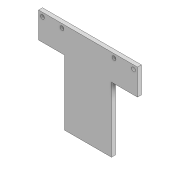
# Autodesk Inventor part: rotator_support
Saved by Autodesk Inventor 2020 (Build 240168000, 168)
## iProperties
Created: 2021-05-10
Part Number: rotator_support
Material: Generic
Document SubType Name: Modeling
Designer: Hsu Daniel
Density: 1 g/cm^3
Appearance: Default
Author: Hsu Daniel
Autodesk Inventor part; units mm, degrees
ref_plane "YZ Plane" through (0, 0, 0) normal (1, 0, 0) x (0, 1, 0)
ref_plane "XZ Plane" through (0, 0, 0) normal (0, 1, 0) x (-1, 0, 0)
ref_plane "XY Plane" through (0, 0, 0) normal (0, 0, 1) x (1, 0, 0)
sketch "Sketch1" plane through (0, 0, 0) normal (0, 0, 1) x (1, 0, 0)
  line L0 (0, 0) -> (0, 50)
  line L1 (0, 50) -> (-20, 50)
  line L2 (-20, 50) -> (-20, 70)
  line L3 (-20, 70) -> (18, 70)
  line L4 (18, 70) -> (18, 0) construction
  line L5 (18, 0) -> (0, 0)
  line L6 (36, 0) -> (36, 50)
  line L7 (36, 50) -> (56, 50)
  line L8 (56, 50) -> (56, 70)
  line L9 (56, 70) -> (18, 70)
  line L10 (18, 0) -> (36, 0)
  circle A0 centre (-17, 67) radius 1.5
  circle A1 centre (-2, 67) radius 1.5
  circle A2 centre (53, 67) radius 1.5
  circle A3 centre (38, 67) radius 1.5
  line L11 (-17, 67) -> (-20, 67) construction
  dimension "d1" = 20
  dimension "d2" = 20
  dimension "d3" = 36
  dimension "d4" = 70
  dimension "d5" = 3
  dimension "d6" = 3
  dimension "d7" = 15
  dimension "d8" = 3
  dimension "d9" = 3
  constraints: 24 end point, 6 perpendicular, 6 symmetric about line, 4 centre point, 2 point on line, 1 vertical, 2 other
  measures "d1" distance of L0.end L1.end
  measures "d2" distance of L1.end L2.end
  measures "d3" distance between parallel lines of L6 L0
  measures "d4" distance between parallel lines of L5 L3
  measures "d5" diameter of A0
  measures "d6" diameter of A1
  measures "d7" distance of A1.centre L11.start
  measures "d8" distance from line of L2 L11.start
  measures "d9" distance from line of L3 L11.start
extrude "Extrusion1" add sketch "Sketch1" along normal blind 3
body "Solid1"
